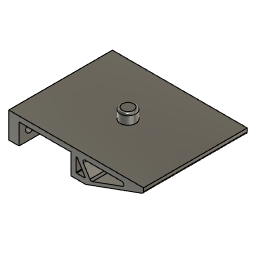
v2.0.0-sim-dash-base (Autodesk Fusion 360 design; units mm, degrees)
Autodesk Fusion 360 part; units mm, degrees
sketch "Sketch1" plane through (0, 0, 0) normal (0, 0, 1) x (1, 0, 0)
  line L0 (-65, 30) -> (65, 30)
  line L1 (65, 30) -> (65, -70)
  line L2 (65, -70) -> (-65, -70)
  line L3 (-65, -70) -> (-65, 30)
  dimension "d1" = 130
  dimension "d2" = 100
  constraint horizontal L0
  constraint vertical L1
  constraint horizontal L2
  constraint vertical L3
  measures "d1" distance of L1.end L2.end
  measures "d2" distance of L0.start L2.end
extrude "Extrude1" add sketch "Sketch1" along normal blind 25
sketch "Sketch3" plane through (-65, 0, 0) normal (-1, 0, 0) x (0, -1, 0)
  line L0 (-30, 0) -> (70, 0)
  line L1 (70, 0) -> (70, 25)
  line L2 (70, 25) -> (-30, 25)
  line L3 (-30, 25) -> (-30, 0)
  circle A0 centre (-20.2556, 10) radius 4
  circle A1 centre (59.7444, 10) radius 4
  dimension "d6" = 8
  dimension "d7" = 10
  dimension "d8" = 80
  constraint equal A0 A1
  constraint horizontal A0.centre A1.centre
  measures "d6" diameter of A0
  measures "d7" distance of L0 A0.centre
  measures "d8" horizontal distance of A0.centre A1.centre
extrude "Extrude2" cut sketch "Sketch3" against normal blind 10 contours A0 | A1
sketch "Sketch4" plane through (0, -70, 0) normal (0, -1, 0) x (1, 0, 0)
  line L0 (-65, 0) -> (65, 0)
  line L1 (65, 0) -> (65, 25)
  line L2 (65, 25) -> (-65, 25)
  line L3 (-65, 25) -> (-65, 0)
  line L4 (-55, 0) -> (-5, 0)
  line L5 (-5, 0) -> (-5, 20)
  line L6 (-5, 20) -> (-55, 20)
  line L7 (-55, 20) -> (-55, 0)
  dimension "d11" = 10
  dimension "d12" = 20
  dimension "d15" = 50
  constraint horizontal L4
  constraint vertical L5
  constraint horizontal L6
  constraint vertical L7
  constraint coincident L0 L4.start
  measures "d11" distance of L3 L7
  measures "d12" distance of L4.start L6.end
  measures "d15" distance of L5.end L6.end
extrude "Extrude3" cut sketch "Sketch4" against normal blind 20 contours L0 L4 L5 L6 L7
sketch "Sketch5" plane through (0, 30, 0) normal (0, 1, 0) x (-1, 0, 0)
  line L0 (-65, 0) -> (65, 0)
  line L1 (65, 0) -> (65, 25)
  line L2 (65, 25) -> (-65, 25)
  line L3 (-65, 25) -> (-65, 0)
  line L4 (5, 20) -> (55, 20)
  line L5 (55, 20) -> (55, 0)
  line L6 (55, 0) -> (5, 0)
  line L7 (5, 0) -> (5, 20)
  dimension "d16" = 50
  dimension "d17" = 20
  dimension "d19" = 10
  constraint horizontal L4
  constraint vertical L5
  constraint horizontal L6
  constraint vertical L7
  constraint coincident L0 L5.end
  measures "d16" distance of L4.start L4.end
  measures "d17" distance of L4.end L5.end
  measures "d19" distance of L1 L5
extrude "Extrude4" cut sketch "Sketch5" against normal blind 20 contours L0 L4 L5 L6 L7
sketch "Sketch6" plane through (0, -70, 0) normal (0, -1, 0) x (1, 0, 0)
  line L0 (-55, 0) -> (-55, 20)
  line L1 (-55, 20) -> (-5, 20)
  line L2 (-5, 20) -> (-5, 0)
  line L3 (-5, 0) -> (65, 0)
  line L4 (65, 0) -> (65, 25)
  line L5 (65, 25) -> (-65, 25)
  line L6 (-65, 25) -> (-65, 0)
  line L7 (-65, 0) -> (-55, 0)
  line L8 (9.1818, 0) -> (65, 20.3162)
  dimension "d22" = 20
  constraint coincident L3 L8.start
  constraint coincident L4 L8.end
  measures "d22" angle of L3 L8
extrude "Extrude5" cut sketch "Sketch6" against normal through all contours L3 L4 L8
sketch "Sketch7" plane through (0, -70, 0) normal (0, -1, 0) x (1, 0, 0)
  line L0 (9.1818, 0) -> (65, 20.3162)
  line L1 (65, 20.3162) -> (65, 25)
  line L2 (65, 25) -> (-65, 25)
  line L3 (-65, 25) -> (-65, 0)
  line L4 (-65, 0) -> (-55, 0)
  line L5 (-55, 0) -> (-55, 20)
  line L6 (-55, 20) -> (-5, 20)
  line L7 (-5, 20) -> (-5, 0)
  line L8 (-5, 0) -> (9.1818, 0)
  line L9 (0, 20) -> (0, 5)
  line L10 (0, 5) -> (9.1818, 5)
  line L11 (9.1818, 5) -> (0, 20)
  line L12 (4.966, 20) -> (55.36, 20)
  line L13 (55.36, 20) -> (14.1478, 5)
  line L14 (14.1478, 5) -> (4.966, 20)
  dimension "d24" = 5
  dimension "d25" = 5
  dimension "d27" = 3
  constraint perpendicular L2 L9
  constraint perpendicular L9 L10
  constraint parallel L2 L12
  constraint parallel L0 L13
  constraint parallel L11 L14
  constraint horizontal L6.end L9.start
  constraint vertical L0.start L10.end
  constraint horizontal L10.end L13.end
  constraint horizontal L9.start L12.start
  measures "d24" distance of L8 L10
  measures "d25" distance of L7 L9
  measures "d27" distance of L0 L13
extrude "Extrude6" cut sketch "Sketch7" against normal through all contours L9 L10 L11 | L12 L13 L14
sketch "Sketch8" plane through (0, -50, 0) normal (0, -1, 0) x (1, 0, 0)
  line L0 (-55, 20) -> (-55, 0)
  line L1 (-55, 0) -> (-5, 0)
  line L2 (-5, 0) -> (-5, 20)
  line L3 (-5, 20) -> (-55, 20)
  line L4 (-45, 20) -> (-30, 5)
  line L5 (-30, 5) -> (-15, 20)
  line L6 (-45, 20) -> (-15, 20)
  dimension "d29" = 45
  dimension "d30" = 45
  dimension "d31" = 5
  constraint coincident L3 L5.end
  constraint parallel L3 L6
  constraint midpoint L3 L6
  measures "d29" angle of L3 L4
  measures "d30" angle of L3 L5
  measures "d31" distance of L1 L4.end
extrude "Extrude7" cut sketch "Sketch8" against normal through all contours L3 L4 L5 L6
sketch "Sketch9" plane through (0, -50, 0) normal (0, -1, 0) x (1, 0, 0)
  line L0 (-30, 5) -> (-45, 20)
  line L1 (-45, 20) -> (-55, 20)
  line L2 (-55, 20) -> (-55, 0)
  line L3 (-55, 0) -> (-5, 0)
  line L4 (-5, 0) -> (-5, 20)
  line L5 (-5, 20) -> (-15, 20)
  line L6 (-15, 20) -> (-30, 5)
  line L7 (-50, 15) -> (-50, 5)
  line L8 (-50, 5) -> (-37.0711, 5)
  line L9 (-37.0711, 5) -> (-47.0711, 15)
  line L10 (-47.0711, 15) -> (-50, 15)
  line L11 (-30, 13.9289) -> (-30, -2.0711)
  line L12 (-12.9289, 15) -> (-10, 15)
  line L13 (-10, 15) -> (-10, 5)
  line L14 (-10, 5) -> (-22.9289, 5)
  line L15 (-22.9289, 5) -> (-12.9289, 15)
  dimension "d33" = 5
  dimension "d34" = 5
  dimension "d35" = 5
  dimension "d36" = 5
  constraint vertical L7
  constraint perpendicular L7 L8
  constraint perpendicular L7 L10
  constraint perpendicular L3 L11
  constraint coincident L0.start L11
  constraint symmetric L7.start L11 L12.end
  constraint symmetric L7.end L11 L13.end
  constraint symmetric L8.end L11 L14.end
  constraint symmetric L9.end L11 L12.start
  measures "d33" distance of L0 L9
  measures "d34" distance of L1 L10
  measures "d35" distance of L2 L7
  measures "d36" distance of L3 L8
extrude "Extrude8" cut sketch "Sketch9" against normal through all contours L7 L8 L9 L10 | L12 L13 L14 L15
sketch "Sketch10" plane through (0, 0, 25) normal (0, 0, 1) x (-1, 0, 0)
  line L0 (65, 70) -> (-65, 70)
  line L1 (-65, 70) -> (-65, -30)
  line L2 (-65, -30) -> (65, -30)
  line L3 (65, -30) -> (65, 70)
  circle A0 centre (0, 20) radius 7.5
  point P0 (0, -30)
  point P1 (65, 20)
  dimension "d38" = 15
  constraint midpoint L2 P0
  constraint vertical A0.centre P0
  constraint midpoint L3 P1
  constraint horizontal A0.centre P1
  measures "d38" diameter of A0
extrude "Extrude9" add sketch "Sketch10" along normal blind 10 contours A0
fillet "Fillet1" radius 2 1 edges at (6.9925, -17.2879, 35)
fillet "Fillet1" radius 2 4 edges at (65, -20, 20.3162) (14.1478, -20, 5) (55.36, -20, 20) (4.966, -20, 20)
fillet "Fillet1" radius 0.5 3 edges at (9.1818, -20, 5) (0, -20, 5) (0, -20, 20)
fillet "Fillet1" radius 0.5 4 edges at (-10, -20, 5) (-10, -20, 15) (-12.9289, -20, 15) (-22.9289, -20, 5)
fillet "Fillet1" radius 0.5 4 edges at (-37.0711, -20, 5) (-50, -20, 5) (-50, -20, 15) (-47.0711, -20, 15)
fillet "Fillet1" radius 2 1 edges at (-30, -20, 5)
